Autodesk Fusion 360 part; units mm, degrees
(part 3 of 4)
sketch "Sketch2" plane through (0, 0, 0) normal (0, 1, 0) x (-1, 0, 0)
  line L0 (13, -8.25) -> (13, -4.1)
  line L1 (13, -4.1) -> (14, -4.1)
  line L2 (13, -4.1) -> (14, -4.1)
  line L3 (14, -4.1) -> (14, -5.1)
  line L4 (14, -5.1) -> (15, -5.1)
  line L5 (15, -5.1) -> (15, -13)
  line L6 (5.1, -15) -> (13, -15)
  line L7 (13, -15) -> (5.1, -15)
  line L8 (5.1, -14) -> (4.1, -14)
  line L9 (4.1, -14) -> (4.1, -13)
  line L10 (4.1, -13) -> (8.25, -13)
  arc A0 (13, -15) -> (15, -13) centre (13, -13) ccw
  line L11 (12.5, -13.5) -> (10.75, -13.5)
  line L12 (9.75, -12.5) -> (9.75, -10.75)
  line L13 (10.75, -9.75) -> (12.5, -9.75)
  line L14 (13.5, -10.75) -> (13.5, -12.5)
  arc A1 (12.5, -13.5) -> (13.5, -12.5) centre (12.5, -12.5) ccw
  line L15 (12.5, -12.5) -> (-13, 13)
  arc A2 (12.5, -13.5) -> (13.5, -12.5) centre (12.5, -12.5) ccw
  arc A3 (9.75, -12.5) -> (10.75, -13.5) centre (10.75, -12.5) ccw
  arc A4 (10.75, -9.75) -> (9.75, -10.75) centre (10.75, -10.75) ccw
  arc A5 (13.5, -10.75) -> (12.5, -9.75) centre (12.5, -10.75) ccw
  line L16 (15, -13) -> (15, -5.1)
  line L17 (12.5, -9.75) -> (10.75, -9.75)
  line L18 (10.75, -13.5) -> (12.5, -13.5)
  line L19 (9.5009, -9.5009) -> (1.6153, -1.6153) construction
  line L20 (8.25, -13) -> (8.25, -9.6642)
  line L21 (8.25, -10.6606) -> (8.25, -13)
  line L22 (13, -8.25) -> (9.6642, -8.25)
  line L23 (5.1, -14) -> (5.1, -15)
  line L24 (9.6642, -8.25) -> (5.5142, -4.1)
  line L25 (8.25, -9.6642) -> (4.1, -5.5142)
  line L26 (13.5, 10.75) -> (13.5, 12.5)
  arc A6 (13.5, 12.5) -> (12.5, 13.5) centre (12.5, 12.5) ccw
  arc A7 (10.75, 13.5) -> (9.75, 12.5) centre (10.75, 12.5) ccw
  line L27 (9.75, 12.5) -> (9.75, 10.75)
  line L28 (9.5009, 9.5009) -> (1.6153, 1.6153) construction
  line L29 (13, 8.25) -> (13, 4.1)
  arc A8 (9.75, 10.75) -> (10.75, 9.75) centre (10.75, 10.75) ccw
  line L30 (13, 4.1) -> (14, 4.1)
  arc A9 (13.5, 12.5) -> (12.5, 13.5) centre (12.5, 12.5) ccw
  line L31 (13, 4.1) -> (14, 4.1)
  line L32 (14, 4.1) -> (14, 5.1)
  line L33 (14, 5.1) -> (15, 5.1)
  line L34 (10.75, 9.75) -> (12.5, 9.75)
  line L35 (12.5, 9.75) -> (10.75, 9.75)
  line L36 (13, 8.25) -> (9.6642, 8.25)
  arc A10 (12.5, 9.75) -> (13.5, 10.75) centre (12.5, 10.75) ccw
  line L37 (4.1, 14) -> (4.1, 13)
  line L38 (5.1, 14) -> (4.1, 14)
  line L39 (15, 13) -> (15, 5.1)
  line L40 (15, 5.1) -> (15, 13)
  line L41 (5.1, 15) -> (13, 15)
  line L42 (13, 15) -> (5.1, 15)
  line L43 (4.1, 13) -> (8.25, 13)
  line L44 (12.5, 13.5) -> (10.75, 13.5)
  line L45 (10.75, 13.5) -> (12.5, 13.5)
  line L46 (8.25, 13) -> (8.25, 9.6642)
  line L47 (9.6642, 8.25) -> (5.5142, 4.1)
  line L48 (8.25, 10.6606) -> (8.25, 13)
  arc A11 (15, 13) -> (13, 15) centre (13, 13) ccw
  line L49 (8.25, 9.6642) -> (4.1, 5.5142)
  line L50 (5.1, 14) -> (5.1, 15)
  line L51 (-8.25, 9.6642) -> (-4.1, 5.5142)
  line L52 (-8.25, 10.6606) -> (-8.25, 13)
  line L53 (-12.5, -13.5) -> (-10.75, -13.5)
  arc A12 (-10.75, 9.75) -> (-9.75, 10.75) centre (-10.75, 10.75) ccw
  line L54 (-8.25, 13) -> (-8.25, 9.6642)
  line L55 (-4.1, -13) -> (-8.25, -13)
  line L56 (-15, -5.1) -> (-15, -13)
  line L57 (-9.75, 12.5) -> (-9.75, 10.75)
  line L58 (-13, -8.25) -> (-13, -4.1)
  line L59 (-8.25, -10.6606) -> (-8.25, -13)
  line L60 (-13, 8.25) -> (-13, 4.1)
  line L61 (-12.5, 13.5) -> (-10.75, 13.5)
  line L62 (-4.1, 13) -> (-8.25, 13)
  line L63 (-4.1, -14) -> (-4.1, -13)
  line L64 (-13, -15) -> (-5.1, -15)
  line L65 (-13.5, 10.75) -> (-13.5, 12.5)
  line L66 (-8.25, -13) -> (-8.25, -9.6642)
  line L67 (-9.6642, 8.25) -> (-5.5142, 4.1)
  arc A13 (-12.5, 13.5) -> (-13.5, 12.5) centre (-12.5, 12.5) ccw
  line L68 (-10.75, 13.5) -> (-12.5, 13.5)
  arc A14 (-13.5, -12.5) -> (-12.5, -13.5) centre (-12.5, -12.5) ccw
  line L69 (-13, -8.25) -> (-9.6642, -8.25)
  arc A15 (-12.5, -9.75) -> (-13.5, -10.75) centre (-12.5, -10.75) ccw
  arc A16 (-10.75, -13.5) -> (-9.75, -12.5) centre (-10.75, -12.5) ccw
  line L70 (-14, 5.1) -> (-15, 5.1)
  line L71 (-14, -5.1) -> (-15, -5.1)
  line L72 (-13, 15) -> (-5.1, 15)
  line L73 (-10.75, 9.75) -> (-12.5, 9.75)
  line L74 (-13, -4.1) -> (-14, -4.1)
  line L75 (-5.1, -14) -> (-5.1, -15)
  line L76 (-14, 4.1) -> (-14, 5.1)
  arc A17 (-9.75, -10.75) -> (-10.75, -9.75) centre (-10.75, -10.75) ccw
  line L77 (-14, -4.1) -> (-14, -5.1)
  line L78 (-15, 13) -> (-15, 5.1)
  line L79 (-10.75, -13.5) -> (-12.5, -13.5)
  line L80 (-13.5, -10.75) -> (-13.5, -12.5)
  line L81 (-5.1, -15) -> (-13, -15)
  arc A18 (-9.75, 12.5) -> (-10.75, 13.5) centre (-10.75, 12.5) ccw
  line L82 (-13, 4.1) -> (-14, 4.1)
  line L83 (-13, -4.1) -> (-14, -4.1)
  line L84 (-5.1, 14) -> (-5.1, 15)
  line L85 (-8.25, -9.6642) -> (-4.1, -5.5142)
  line L86 (-13, 4.1) -> (-14, 4.1)
  arc A19 (-13.5, 10.75) -> (-12.5, 9.75) centre (-12.5, 10.75) ccw
  line L87 (-15, -13) -> (-15, -5.1)
  line L88 (-9.5009, 9.5009) -> (-1.6152, 1.6153) construction
  line L89 (-10.75, -9.75) -> (-12.5, -9.75)
  line L90 (-5.1, 14) -> (-4.1, 14)
  line L91 (-15, 5.1) -> (-15, 13)
  line L92 (-9.75, -12.5) -> (-9.75, -10.75)
  arc A20 (-13, 15) -> (-15, 13) centre (-13, 13) ccw
  line L93 (-12.5, -9.75) -> (-10.75, -9.75)
  arc A21 (-15, -13) -> (-13, -15) centre (-13, -13) ccw
  arc A22 (-13.5, -12.5) -> (-12.5, -13.5) centre (-12.5, -12.5) ccw
  arc A23 (-12.5, 13.5) -> (-13.5, 12.5) centre (-12.5, 12.5) ccw
  line L94 (-5.1, -14) -> (-4.1, -14)
  line L95 (-12.5, 9.75) -> (-10.75, 9.75)
  line L96 (-9.5009, -9.5009) -> (-1.6152, -1.6153) construction
  line L97 (-5.1, 15) -> (-13, 15)
  line L98 (-13, 8.25) -> (-9.6642, 8.25)
  line L99 (-9.6642, -8.25) -> (-5.5142, -4.1)
  line L100 (-4.1, 14) -> (-4.1, 13)
  line L101 (4.1, -5.5142) -> (-4.1, -5.5142)
  line L102 (5.5142, 4.1) -> (5.5142, -4.1)
  line L103 (-5.5142, 4.1) -> (-5.5142, -4.1)
  line L104 (4.1, 5.5142) -> (-4.1, 5.5142)
  circle A24 centre (0, 0) radius 3.4
  point P0 (13, -8.25)
  point P1 (14, -4.1)
  point P2 (14, -5.1)
  point P3 (15, -5.1)
  point P4 (15, -15)
  point P5 (5.1, -15)
  point P6 (5.1, -14)
  point P7 (4.1, -14)
  point P8 (4.1, -13)
  point P9 (8.25, -13)
  point P10 (0, 0)
  point P11 (15, 0)
  point P12 (0, 15)
  point P13 (0, 0)
  point P14 (15, 15)
  point P15 (12.5, 12.5)
  point P16 (5.1, 14)
  point P17 (5.1, 15)
  point P18 (8.25, 13)
  point P19 (4.1, 13)
  point P20 (14, 5.1)
  point P21 (4.1, 14)
  point P22 (14, 4.1)
  point P23 (13, 8.25)
  point P24 (15, 5.1)
  point P25 (-12.5, 12.5)
  point P26 (-15, 0)
  point P27 (-5.1, 15)
  point P28 (-8.25, 13)
  point P29 (-4.1, 13)
  point P30 (-5.1, -15)
  point P31 (-15, 15)
  point P32 (-14, 5.1)
  point P33 (-4.1, 14)
  point P34 (-14, 4.1)
  point P35 (-13, 8.25)
  point P36 (-15, 5.1)
  point P37 (-4.1, -13)
  point P38 (0, 0)
  point P39 (0, 0)
  point P40 (0, 15)
  point P41 (0, 15)
  point P42 (0, -15)
  point P43 (0, 0)
  point P44 (-8.25, -13)
  point P45 (-4.1, -14)
  point P46 (-15, -15)
  point P47 (-5.1, -14)
  point P48 (-12.5, -12.5)
  point P49 (0, 0)
  point P50 (-5.1, 14)
  point P51 (-15, -5.1)
  point P52 (-14, -5.1)
  point P53 (-13, -8.25)
  point P54 (-14, -4.1)
  point P55 (-15, 0)
  dimension "d78" = 2
  dimension "d79" = 1
  dimension "d80" = 1.5
  dimension "d91" = 1
  dimension "d92" = 1
  dimension "d93" = 1.5
  dimension "d94" = 1.5
  dimension "d102" = 3.75
  dimension "d103" = 1.5
  dimension "d104" = 3.75
  dimension "d105" = 2
  dimension "d106" = 2
  dimension "d109" = 5.869
  dimension "d110" = 5.869
  dimension "d111" = 3.3358
  dimension "d112" = 3.3358
  dimension "d113" = 4.15
  dimension "d114" = 4.15
  dimension "d115" = 8.2
  dimension "d116" = 8.2
  dimension "d117" = 8.2
  dimension "d118" = 8.2
  dimension "d119" = 6.8
  constraint coincident L0.end L1.start
  constraint coincident P1 L1.end
  constraint coincident P2 L3.end
  constraint coincident P3 L4.end
  constraint coincident P5 L6.start
  constraint coincident P6 L8.start
  constraint coincident P7 L8.end
  constraint coincident P8 L9.end
  constraint coincident P9 L10.end
  constraint tangent L5 A0
  constraint tangent L7 A0
  constraint horizontal L11
  constraint vertical L12
  constraint horizontal L13
  constraint vertical L14
  constraint tangent L14 A2
  constraint tangent L11 A2
  constraint tangent L11 A3
  constraint tangent L12 A3
  constraint equal A2 A3
  constraint tangent L12 A4
  constraint tangent L13 A4
  constraint equal A2 A4
  constraint tangent L13 A5
  constraint tangent L14 A5
  constraint equal A2 A5
  constraint coincident L15 L19.start
  constraint coincident L15 L19.end
  constraint parallel L15 L19
  constraint perpendicular L10 L20
  constraint coincident P0 L0.start
  constraint perpendicular L0 L22
  constraint parallel L19 L24
  constraint parallel L19 L25
  constraint perpendicular L7 L23
  constraint coincident P49 P43
  measures "d78" radius of A0
  measures "d79" radius of A2
  measures "d80" distance of L14 L16
  measures "d91" distance of L19 L24
  measures "d92" distance of L15 L25
  measures "d93" distance of L12 L20
  measures "d94" distance of L13 L22
  measures "d102" distance of L12 L14
  measures "d103" distance of L7 L11
  measures "d104" distance of L11 L13
  measures "d105" distance of L7 L10
  measures "d106" distance of L0 L5
  measures "d109" distance of L22.end L24.end
  measures "d110" distance of L20.end L25.end
  measures "d111" distance of P9 L20.end
  measures "d112" distance of P0 L22.end
  measures "d113" distance of P8 P9
  measures "d114" distance of P0 L0.end
  measures "d115" distance of L25.end L85.end
  measures "d116" distance of L24.end L47.end
  measures "d117" distance of L67.end L99.end
  measures "d118" distance of L49.end L51.end
  measures "d119" diameter of A24
extrude "Extrude1" add sketch "Sketch2" along normal blind 100
move_body "Move1" bodies 1 to x (0, -1, 0) y (1, 0, 0) z (0, 0, 1) at (-3.4, 15.1, 15)
move_body "Move2" bodies 1 to x (1, 0, 0) y (0, 1, 0) z (0, 0, 1) at (3.4, 0, 0)
sketch "Sketch3" plane through (0, 0, 30) normal (0, 0, 1) x (1, 0, 0)
  line L0 (0, 10) -> (0, 2.1)
  line L1 (0, 2.1) -> (100, 2.1)
  line L2 (100, 2.1) -> (100, 10)
  line L3 (100, 10) -> (0, 10)
  line L4 (0, 0) -> (64.1772, 37.0527)
  line L5 (0, 0) -> (74.1054, 0) construction
  line L6 (64.1772, 37.0527) -> (-5, 37.0527)
  line L7 (-5, 37.0527) -> (-5, 0)
  line L8 (-5, 0) -> (0, 0)
  line L9 (100, 30) -> (54.3421, 30) construction
  line L10 (100, 0) -> (78.7466, 36.812)
  line L11 (100, 0) -> (57.4932, 0) construction
  line L12 (78.7466, 36.812) -> (120, 36.812)
  line L13 (120, 36.812) -> (120, -10)
  line L14 (120, -10) -> (99.3733, -10)
  line L15 (99.3733, -10) -> (100, 0)
  dimension "d122" = 30
  dimension "d126" = 60
  constraint horizontal L5
  constraint coincident L4.start L5.start
  constraint horizontal L6
  constraint perpendicular L6 L7
  constraint perpendicular L7 L8
  constraint horizontal L9
  constraint horizontal L11
  constraint parallel L3 L12
  constraint perpendicular L3 L13
  constraint perpendicular L13 L14
  measures "d122" angle of L4 L5
  measures "d126" angle of L10 L11
extrude "Extrude2" cut sketch "Sketch3" against normal blind 60 contours L0 L1 L3 L4 | L0 L1 L3 L4 L6 L7 L8 | L1 L2 L3 L10 L12 L13 L14 L15 | L1 L2 L3 L10
equation "d33 = ( 8.2 / 2 ) * 1 mm"
equation "d59 = ( 8.5 / 2 ) * 1 mm"
equation "d60 = ( 8.5 / 2 ) * 1 mm"
equation "d72 = ( 8.2 / 2 ) * 1 mm"
equation "Length = 100 mm"

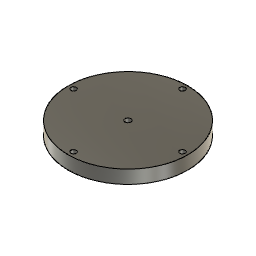
design "lidar_holder"
Autodesk Fusion 360 part; units mm, degrees
sketch "Sketch1" plane through (0, 0, 0) normal (0, 0, 1) x (1, 0, 0)
  circle A0 centre (0, 0) radius 45
  circle A1 centre (-41, 0) radius 2
  circle A2 centre (0, -41) radius 2
  circle A3 centre (41, 0) radius 2
  circle A4 centre (0, 41) radius 2
  circle A5 centre (0, 0) radius 2.25
  dimension "d1" = 90
  dimension "d2" = 4
  dimension "d4" = 4
  dimension "d5" = 4
  dimension "d6" = 4
  dimension "d7" = 4.5
  constraint coincident A0.centre A5.centre
  measures "d1" diameter of A0
  measures "d2" diameter of A1
  measures "d4" diameter of A2
  measures "d5" diameter of A3
  measures "d6" diameter of A4
  measures "d7" diameter of A5
extrude "Extrude1" add sketch "Sketch1" along normal blind 10

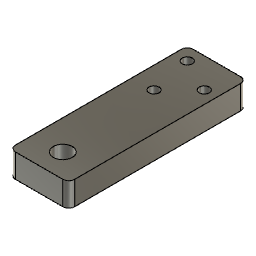
design "wheel_holder"
Autodesk Fusion 360 part; units mm, degrees
sketch "Sketch1" plane through (0, 0, 0) normal (0, 0, 1) x (1, 0, 0)
  line L0 (0, 0) -> (50, 0)
  line L1 (50, 0) -> (50, 150)
  line L2 (50, 150) -> (0, 150)
  line L3 (0, 150) -> (0, 0)
  dimension "d1" = 150
  dimension "d2" = 50
  constraint horizontal L0
  constraint vertical L1
  constraint horizontal L2
  constraint vertical L3
  constraint coincident L0.start L3.end
  measures "d1" distance of L0.start L2.end
  measures "d2" distance of L0.start L0.end
extrude "Extrude1" add sketch "Sketch1" along normal blind 20
fillet "Fillet1" radius 5 4 edges at (0, 0, 10) (50, 0, 10) (50, 150, 10) (0, 150, 10)
sketch "Sketch2" plane through (0, 0, 20) normal (0, 0, 1) x (-1, 0, 0)
  arc A0 (-5, -150) -> (0, -145) centre (-5, -145) ccw
  line L0 (0, -145) -> (0, -5)
  arc A1 (0, -5) -> (-5, 0) centre (-5, -5) ccw
  line L1 (-5, 0) -> (-45, 0)
  arc A2 (-45, 0) -> (-50, -5) centre (-45, -5) ccw
  line L2 (-50, -5) -> (-50, -145)
  arc A3 (-50, -145) -> (-45, -150) centre (-45, -145) ccw
  line L3 (-45, -150) -> (-5, -150)
  circle A4 centre (-25, -20) radius 8
  circle A5 centre (-39.3934, -125) radius 4.25
  circle A6 centre (-18.1802, -103.8009) radius 4.25
  circle A7 centre (-11.0104, -138.9896) radius 4.25
  dimension "d6" = 16
  dimension "d7" = 20
  dimension "d10" = 8.5
  dimension "d13" = 8.5
  dimension "d19" = 8.5
  dimension "d26" = 8.5
  measures "d6" diameter of A4
  measures "d7" distance of L1 A4.centre
  measures "d10" diameter of A5
  measures "d13" diameter of A6
  measures "d19" diameter of A7
  measures "d26" distance of A0.centre A7.centre
extrude "Extrude2" cut sketch "Sketch2" against normal blind 60 contours A4 | A5 | A6 | A7

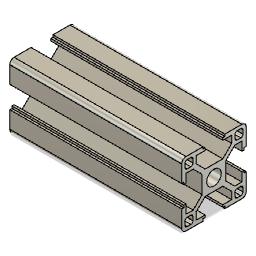
design "tslot_80mm"
Autodesk Fusion 360 part; units mm, degrees
sketch "Sketch1" plane through (0, 0, 0) normal (0, 1, 0) x (1, 0, 0)
  circle A0 centre (0, 0) radius 3.4
  line L0 (5.8, -4.25) -> (5.8, 4.25)
  line L1 (4.4302, 5.8) -> (-4.0698, 5.8)
  line L2 (-5.8, 4.25) -> (-5.8, -4.25)
  arc A1 (-13, 15) -> (-15, 13) centre (-13, 13) ccw
  arc A2 (15, 13) -> (13, 15) centre (13, 13) ccw
  arc A3 (12.9984, -15) -> (15, -13) centre (13, -13) ccw
  arc A4 (-15, -13.001) -> (-13, -15) centre (-13, -13) ccw
  line L3 (-9.0785, 8.25) -> (-13, 8.25)
  line L4 (-10.4448, -8.25) -> (-13, -8.25)
  line L5 (-8.25, 10.6606) -> (-8.25, 13)
  line L6 (8.25, 9.241) -> (8.25, 13)
  line L7 (-12.5, 9.75) -> (-10.75, 9.75)
  line L8 (-9.75, 10.75) -> (-9.75, 12.5)
  line L9 (-10.75, 13.5) -> (-12.5, 13.5)
  line L10 (-13.5, 12.5) -> (-13.5, 10.75)
  arc A5 (-12.5, 13.5) -> (-13.5, 12.5) centre (-12.5, 12.5) ccw
  arc A6 (-9.75, 12.5) -> (-10.75, 13.5) centre (-10.75, 12.5) ccw
  arc A7 (-10.75, 9.75) -> (-9.75, 10.75) centre (-10.75, 10.75) ccw
  arc A8 (-13.5, 10.75) -> (-12.5, 9.75) centre (-12.5, 10.75) ccw
  line L11 (-4.1, 14) -> (-5.1, 14)
  line L12 (-5.1, 14) -> (-5.1, 15)
  line L13 (4.1, 13) -> (4.1, 14)
  line L14 (4.1, 14) -> (5.1, 14)
  line L15 (5.1, 14) -> (5.1, 15)
  line L16 (-4.1, 14) -> (-4.1, 13)
  line L17 (0, 15) -> (0, -15) construction
  line L18 (-15, 0) -> (15, 0) construction
  line L19 (13.5, 12.5) -> (13.5, 10.75)
  line L20 (12.5, 9.75) -> (10.75, 9.75)
  arc A9 (10.75, 13.5) -> (9.75, 12.5) centre (10.75, 12.5) ccw
  arc A10 (9.75, 10.75) -> (10.75, 9.75) centre (10.75, 10.75) ccw
  line L21 (9.75, 10.75) -> (9.75, 12.5)
  arc A11 (12.5, 9.75) -> (13.5, 10.75) centre (12.5, 10.75) ccw
  line L22 (10.75, 13.5) -> (12.5, 13.5)
  arc A12 (13.5, 12.5) -> (12.5, 13.5) centre (12.5, 12.5) ccw
  arc A13 (-9.75, -10.75) -> (-10.75, -9.75) centre (-10.75, -10.75) ccw
  line L23 (-9.75, -10.75) -> (-9.75, -12.5)
  line L24 (-13.5, -12.5) -> (-13.5, -10.75)
  line L25 (-10.75, -13.5) -> (-12.5, -13.5)
  arc A14 (-13.5, -12.5) -> (-12.5, -13.5) centre (-12.5, -12.5) ccw
  line L26 (-12.5, -9.75) -> (-10.75, -9.75)
  arc A15 (-12.5, -9.75) -> (-13.5, -10.75) centre (-12.5, -10.75) ccw
  arc A16 (-10.75, -13.5) -> (-9.75, -12.5) centre (-10.75, -12.5) ccw
  arc A17 (12.5, -13.5) -> (13.5, -12.5) centre (12.5, -12.5) ccw
  arc A18 (10.75, -9.75) -> (9.75, -10.75) centre (10.75, -10.75) ccw
  arc A19 (9.75, -12.5) -> (10.75, -13.5) centre (10.75, -12.5) ccw
  line L27 (9.75, -10.75) -> (9.75, -12.5)
  line L28 (12.5, -9.75) -> (10.75, -9.75)
  arc A20 (13.5, -10.75) -> (12.5, -9.75) centre (12.5, -10.75) ccw
  line L29 (13.5, -12.5) -> (13.5, -10.75)
  line L30 (10.75, -13.5) -> (12.5, -13.5)
  line L31 (-4.1, -14) -> (-5.1, -14)
  line L32 (-4.1, -14) -> (-4.1, -13)
  line L33 (-5.1, -14) -> (-5.1, -15)
  line L34 (4.1, -13) -> (4.1, -14)
  line L35 (4.1, -14) -> (5.1, -14)
  line L36 (5.1, -14) -> (5.1, -15)
  line L37 (-8.25, -10.6606) -> (-8.25, -13)
  line L38 (-13, -15) -> (-5.1, -15)
  line L39 (5.1, -15) -> (12.9984, -15)
  line L40 (-8.25, -13) -> (-4.1, -13)
  line L41 (13, 15) -> (5.1, 15)
  line L42 (-5.1, 15) -> (-13, 15)
  line L43 (8.25, 13) -> (4.1, 13)
  line L44 (-4.1, 13) -> (-8.25, 13)
  line L45 (8.25, -9.768) -> (8.25, -13)
  line L46 (-13, -13) -> (12.5, 12.5) construction
  line L47 (-12.5, 12.5) -> (13, -13) construction
  line L48 (13, -8.25) -> (9.8438, -8.25)
  line L49 (5.8, -4.25) -> (9.8438, -8.25)
  line L50 (4.1, -13) -> (8.25, -13)
  line L51 (13, 8.25) -> (9.3051, 8.25)
  line L52 (-4.2601, -5.7908) -> (4.2399, -5.7908)
  line L53 (-13, 4.1) -> (-14, 4.1)
  line L54 (-14, 4.1) -> (-14, 5.1)
  line L55 (-14, 5.1) -> (-15, 5.1)
  line L56 (-13, -4.1) -> (-14, -4.1)
  line L57 (-14, -4.1) -> (-14, -5.1)
  line L58 (-14, -5.1) -> (-15, -5.1)
  line L59 (-13, 8.25) -> (-13, 4.1)
  line L60 (-13, -4.1) -> (-13, -8.25)
  line L61 (-15, 13) -> (-15, 5.1)
  line L62 (-15, -5.1) -> (-15, -13.001)
  line L63 (13, -8.25) -> (13, -3.9838)
  line L64 (13, 4.0895) -> (13, 10.5589)
  line L65 (15, -13) -> (15, -4.9838)
  line L66 (15, 5.0895) -> (15, 13)
  point P0 (15, -15)
  point P1 (15, 15)
  point P2 (-15, 15)
  point P3 (13, 13)
  point P4 (-13, -13)
  point P5 (13, -13)
  point P6 (13, -13)
  point P7 (13, -10.5589)
  dimension "d1" = 6.8
  dimension "d2" = 30
  dimension "d3" = 30
  dimension "d5" = 9.2
  dimension "d6" = 9.2
  dimension "d7" = 9.2
  dimension "d13" = 2
  dimension "d14" = 2
  dimension "d15" = 2
  dimension "d16" = 2
  dimension "d17" = 16.5
  dimension "d19" = 16.5
  dimension "d22" = 1.5
  dimension "d23" = 1.5
  dimension "d24" = 1.5
  dimension "d25" = 1.5
  dimension "d26" = 1
  dimension "d33" = 4.1
  dimension "d34" = 1
  dimension "d35" = 2
  dimension "d36" = 2
  dimension "d37" = 2
  dimension "d39" = 3.75
  dimension "d40" = 3.75
  dimension "d41" = 5.8
  dimension "d42" = 5.8
  dimension "d43" = 5.8
  dimension "d45" = 8.5
  dimension "d46" = 8.5
  dimension "d48" = 8.5
  dimension "d49" = 1
  dimension "d51" = 8.2
  dimension "d52" = 1.5
  dimension "d53" = 1.5
  dimension "d54" = 1.5
  dimension "d55" = 1.5
  dimension "d57" = 1.5
  dimension "d58" = 1.5
  dimension "d59" = 4.25
  dimension "d60" = 4.25
  dimension "d64" = 8.5
  dimension "d65" = 1
  dimension "d66" = 1
  dimension "d67" = 1
  dimension "d68" = 1
  dimension "d71" = 8.2
  dimension "d72" = 4.1
  constraint horizontal L38
  constraint vertical L65
  constraint horizontal L41
  constraint vertical L61
  constraint vertical L0
  constraint horizontal L1
  constraint vertical L2
  constraint coincident P2 L61
  constraint coincident P2 L41
  constraint tangent A1 L61
  constraint coincident P1 L41
  constraint coincident P1 L65
  constraint tangent A2 L41
  constraint coincident P0 L38
  constraint coincident P0 L65
  constraint tangent A3 L65
  constraint tangent A4 L38
  constraint parallel L63 L65
  constraint horizontal L7
  constraint vertical L8
  constraint horizontal L9
  constraint vertical L10
  constraint tangent L10 A5
  constraint tangent L9 A5
  constraint tangent L9 A6
  constraint tangent L8 A6
  constraint equal A5 A6
  constraint tangent L8 A7
  constraint tangent L7 A7
  constraint equal A5 A7
  constraint tangent L7 A8
  constraint tangent L10 A8
  constraint equal A5 A8
  constraint perpendicular L12 L41
  constraint perpendicular L13 L43
  constraint perpendicular L13 L14
  constraint perpendicular L15 L41
  constraint coincident L16.end L43
  constraint perpendicular L16 L43
  constraint symmetric A1.centre L17 P3
  constraint symmetric L10.start L17 L19.start
  constraint symmetric L9.end L17 L22.end
  constraint symmetric A5 L17 A12
  constraint symmetric L9.start L17 A9.start
  constraint symmetric L8.end L17 A9.end
  constraint symmetric A6 L17 A9
  constraint symmetric L8.start L17 A10.start
  constraint symmetric L7.end L17 L20.end
  constraint symmetric A7 L17 A10
  constraint symmetric L7.start L17 L20.start
  constraint symmetric L10.end L17 L19.end
  constraint symmetric A8 L17 A11
  constraint symmetric P3 L18 P6
  constraint symmetric L64.end L18 P7
  constraint symmetric L18 L19.end A20.start
  constraint symmetric L18 L20.end A18.start
  constraint symmetric L18 P3 P6
  constraint symmetric L18 L19.start A17.end
  constraint symmetric L18 L22.end A17.start
  constraint symmetric L18 A9.end A19.start
  constraint symmetric L18 L20.start L28.start
  constraint symmetric L18 A10.start A18.end
  constraint symmetric L18 A9.start A19.end
  constraint symmetric L18 A9 A19
  constraint symmetric L18 A10 A18
  constraint symmetric L18 A11 A20
  constraint symmetric L18 A12 A17
  constraint symmetric L5.end L18 L37.end
  constraint symmetric L11.start L18 L31.start
  constraint symmetric L11.end L18 L31.end
  constraint symmetric L12.end L18 L33.end
  constraint symmetric L13.start L18 L34.start
  constraint symmetric L13.end L18 L34.end
  constraint symmetric L14.end L18 L35.end
  constraint symmetric L15.end L18 L36.end
  constraint symmetric L16.end L18 L32.end
  constraint collinear L38 L39
  constraint collinear L41 L42
  constraint collinear L43 L44
  constraint symmetric L17 L37.end L45.end
  constraint coincident P4 A4.centre
  constraint coincident A12.centre L46.end
  constraint coincident A5.centre L47.start
  constraint coincident P6 P5
  constraint perpendicular L48 L63
  constraint vertical L45
  constraint coincident L51.start L63
  constraint horizontal L52
  constraint coincident L56.start L59
  constraint coincident L58.end L61
  constraint collinear L59 L60
  constraint collinear L61 L62
  constraint perpendicular L53 L54
  constraint perpendicular L54 L55
  constraint perpendicular L57 L58
  constraint perpendicular L56 L57
  constraint perpendicular L58 L62
  constraint collinear L65 L66
  measures "d1" diameter of A0
  measures "d2" distance of P0 P1
  measures "d3" distance of P1 P2
  measures "d5" distance of L0 L65
  measures "d6" distance of L2 L61
  measures "d7" distance of L1 L41
  measures "d13" radius of A1
  measures "d14" radius of A2
  measures "d15" radius of A3
  measures "d16" radius of A4
  measures "d17" distance of L3 L4
  measures "d19" distance of L5 L6
  measures "d22" distance of L5 L8
  measures "d23" distance of L10 L61
  measures "d24" distance of L3 L7
  measures "d25" distance of L9 L41
  measures "d26" radius of A5
  measures "d33" distance of A0.centre L13
  measures "d34" distance of L11.start L11.end
  measures "d35" distance of L41 L43
  measures "d36" distance of L59 L61
  measures "d37" distance of L63 L65
  measures "d39" distance of L8 L10
  measures "d40" distance of L7 L9
  measures "d41" distance of A0.centre L1
  measures "d42" distance of A0.centre L2
  measures "d43" distance of A0.centre L0
  measures "d45" distance of L1.end L1.start
  measures "d46" distance of L2.start L2.end
  measures "d48" distance of L0.start L0.end
  measures "d49" distance of L13.end L14.end
  measures "d51" distance of L13 L16
  measures "d52" distance of L23 L37
  measures "d53" distance of L4 L26
  measures "d54" distance of L27 L45
  measures "d55" distance of L28 L48
  measures "d57" distance of L20 L51
  measures "d58" distance of L6 L21
  measures "d59" distance of L2.end L18
  measures "d60" distance of L0.start L18
  measures "d64" distance of L52.start L52.end
  measures "d65" distance of L53.end L54.end
  measures "d66" distance of L53.start L53.end
  measures "d67" distance of L56.start L56.end
  measures "d68" distance of L56.end L57.end
  measures "d71" distance of L53 L56
  measures "d72" distance of L18 L53
sketch "Sketch2" plane through (0, 0, 0) normal (0, 1, 0) x (-1, 0, 0)
  line L0 (13, -8.25) -> (13, -4.1)
  line L1 (13, -4.1) -> (14, -4.1)
  line L2 (13, -4.1) -> (14, -4.1)
  line L3 (14, -4.1) -> (14, -5.1)
  line L4 (14, -5.1) -> (15, -5.1)
  line L5 (15, -5.1) -> (15, -13)
  line L6 (5.1, -15) -> (13, -15)
  line L7 (13, -15) -> (5.1, -15)
  line L8 (5.1, -14) -> (4.1, -14)
  line L9 (4.1, -14) -> (4.1, -13)
  line L10 (4.1, -13) -> (8.25, -13)
  arc A0 (13, -15) -> (15, -13) centre (13, -13) ccw
  line L11 (12.5, -13.5) -> (10.75, -13.5)
  line L12 (9.75, -12.5) -> (9.75, -10.75)
  line L13 (10.75, -9.75) -> (12.5, -9.75)
  line L14 (13.5, -10.75) -> (13.5, -12.5)
  arc A1 (12.5, -13.5) -> (13.5, -12.5) centre (12.5, -12.5) ccw
  line L15 (12.5, -12.5) -> (-13, 13)
  arc A2 (12.5, -13.5) -> (13.5, -12.5) centre (12.5, -12.5) ccw
  arc A3 (9.75, -12.5) -> (10.75, -13.5) centre (10.75, -12.5) ccw
  arc A4 (10.75, -9.75) -> (9.75, -10.75) centre (10.75, -10.75) ccw
  arc A5 (13.5, -10.75) -> (12.5, -9.75) centre (12.5, -10.75) ccw
  line L16 (15, -13) -> (15, -5.1)
  line L17 (12.5, -9.75) -> (10.75, -9.75)
  line L18 (10.75, -13.5) -> (12.5, -13.5)
  line L19 (9.5009, -9.5009) -> (1.6153, -1.6153) construction
  line L20 (8.25, -13) -> (8.25, -9.6642)
  line L21 (8.25, -10.6606) -> (8.25, -13)
  line L22 (13, -8.25) -> (9.6642, -8.25)
  line L23 (5.1, -14) -> (5.1, -15)
  line L24 (9.6642, -8.25) -> (5.5142, -4.1)
  line L25 (8.25, -9.6642) -> (4.1, -5.5142)
  line L26 (13.5, 10.75) -> (13.5, 12.5)
  arc A6 (13.5, 12.5) -> (12.5, 13.5) centre (12.5, 12.5) ccw
  arc A7 (10.75, 13.5) -> (9.75, 12.5) centre (10.75, 12.5) ccw
  line L27 (9.75, 12.5) -> (9.75, 10.75)
  line L28 (9.5009, 9.5009) -> (1.6153, 1.6153) construction
  line L29 (13, 8.25) -> (13, 4.1)
  arc A8 (9.75, 10.75) -> (10.75, 9.75) centre (10.75, 10.75) ccw
  line L30 (13, 4.1) -> (14, 4.1)
  arc A9 (13.5, 12.5) -> (12.5, 13.5) centre (12.5, 12.5) ccw
  line L31 (13, 4.1) -> (14, 4.1)
  line L32 (14, 4.1) -> (14, 5.1)
  line L33 (14, 5.1) -> (15, 5.1)
  line L34 (10.75, 9.75) -> (12.5, 9.75)
  line L35 (12.5, 9.75) -> (10.75, 9.75)
  line L36 (13, 8.25) -> (9.6642, 8.25)
  arc A10 (12.5, 9.75) -> (13.5, 10.75) centre (12.5, 10.75) ccw
  line L37 (4.1, 14) -> (4.1, 13)
  line L38 (5.1, 14) -> (4.1, 14)
  line L39 (15, 13) -> (15, 5.1)
  line L40 (15, 5.1) -> (15, 13)
  line L41 (5.1, 15) -> (13, 15)
  line L42 (13, 15) -> (5.1, 15)
  line L43 (4.1, 13) -> (8.25, 13)
  line L44 (12.5, 13.5) -> (10.75, 13.5)
  line L45 (10.75, 13.5) -> (12.5, 13.5)
  line L46 (8.25, 13) -> (8.25, 9.6642)
  line L47 (9.6642, 8.25) -> (5.5142, 4.1)
  line L48 (8.25, 10.6606) -> (8.25, 13)
  arc A11 (15, 13) -> (13, 15) centre (13, 13) ccw
  line L49 (8.25, 9.6642) -> (4.1, 5.5142)
  line L50 (5.1, 14) -> (5.1, 15)
  line L51 (-8.25, 9.6642) -> (-4.1, 5.5142)
  line L52 (-8.25, 10.6606) -> (-8.25, 13)
  line L53 (-12.5, -13.5) -> (-10.75, -13.5)
  arc A12 (-10.75, 9.75) -> (-9.75, 10.75) centre (-10.75, 10.75) ccw
  line L54 (-8.25, 13) -> (-8.25, 9.6642)
  line L55 (-4.1, -13) -> (-8.25, -13)
  line L56 (-15, -5.1) -> (-15, -13)
  line L57 (-9.75, 12.5) -> (-9.75, 10.75)
  line L58 (-13, -8.25) -> (-13, -4.1)
  line L59 (-8.25, -10.6606) -> (-8.25, -13)
  line L60 (-13, 8.25) -> (-13, 4.1)
  line L61 (-12.5, 13.5) -> (-10.75, 13.5)
  line L62 (-4.1, 13) -> (-8.25, 13)
  line L63 (-4.1, -14) -> (-4.1, -13)
  line L64 (-13, -15) -> (-5.1, -15)
  line L65 (-13.5, 10.75) -> (-13.5, 12.5)
  line L66 (-8.25, -13) -> (-8.25, -9.6642)
  line L67 (-9.6642, 8.25) -> (-5.5142, 4.1)
  arc A13 (-12.5, 13.5) -> (-13.5, 12.5) centre (-12.5, 12.5) ccw
  line L68 (-10.75, 13.5) -> (-12.5, 13.5)
  arc A14 (-13.5, -12.5) -> (-12.5, -13.5) centre (-12.5, -12.5) ccw
  line L69 (-13, -8.25) -> (-9.6642, -8.25)
  arc A15 (-12.5, -9.75) -> (-13.5, -10.75) centre (-12.5, -10.75) ccw
  arc A16 (-10.75, -13.5) -> (-9.75, -12.5) centre (-10.75, -12.5) ccw
  line L70 (-14, 5.1) -> (-15, 5.1)
  line L71 (-14, -5.1) -> (-15, -5.1)
  line L72 (-13, 15) -> (-5.1, 15)
  line L73 (-10.75, 9.75) -> (-12.5, 9.75)
  line L74 (-13, -4.1) -> (-14, -4.1)
  line L75 (-5.1, -14) -> (-5.1, -15)
  line L76 (-14, 4.1) -> (-14, 5.1)
  arc A17 (-9.75, -10.75) -> (-10.75, -9.75) centre (-10.75, -10.75) ccw
  line L77 (-14, -4.1) -> (-14, -5.1)
  line L78 (-15, 13) -> (-15, 5.1)
  line L79 (-10.75, -13.5) -> (-12.5, -13.5)
  line L80 (-13.5, -10.75) -> (-13.5, -12.5)
  line L81 (-5.1, -15) -> (-13, -15)
  arc A18 (-9.75, 12.5) -> (-10.75, 13.5) centre (-10.75, 12.5) ccw
  line L82 (-13, 4.1) -> (-14, 4.1)
  line L83 (-13, -4.1) -> (-14, -4.1)
  line L84 (-5.1, 14) -> (-5.1, 15)
  line L85 (-8.25, -9.6642) -> (-4.1, -5.5142)
  line L86 (-13, 4.1) -> (-14, 4.1)
  arc A19 (-13.5, 10.75) -> (-12.5, 9.75) centre (-12.5, 10.75) ccw
  line L87 (-15, -13) -> (-15, -5.1)
  line L88 (-9.5009, 9.5009) -> (-1.6152, 1.6153) construction
  line L89 (-10.75, -9.75) -> (-12.5, -9.75)
  line L90 (-5.1, 14) -> (-4.1, 14)
  line L91 (-15, 5.1) -> (-15, 13)
  line L92 (-9.75, -12.5) -> (-9.75, -10.75)
  arc A20 (-13, 15) -> (-15, 13) centre (-13, 13) ccw
  line L93 (-12.5, -9.75) -> (-10.75, -9.75)
  arc A21 (-15, -13) -> (-13, -15) centre (-13, -13) ccw
  arc A22 (-13.5, -12.5) -> (-12.5, -13.5) centre (-12.5, -12.5) ccw
  arc A23 (-12.5, 13.5) -> (-13.5, 12.5) centre (-12.5, 12.5) ccw
  line L94 (-5.1, -14) -> (-4.1, -14)
  line L95 (-12.5, 9.75) -> (-10.75, 9.75)
  line L96 (-9.5009, -9.5009) -> (-1.6152, -1.6153) construction
  line L97 (-5.1, 15) -> (-13, 15)
  line L98 (-13, 8.25) -> (-9.6642, 8.25)
  line L99 (-9.6642, -8.25) -> (-5.5142, -4.1)
  line L100 (-4.1, 14) -> (-4.1, 13)
  line L101 (4.1, -5.5142) -> (-4.1, -5.5142)
  line L102 (5.5142, 4.1) -> (5.5142, -4.1)
  line L103 (-5.5142, 4.1) -> (-5.5142, -4.1)
  line L104 (4.1, 5.5142) -> (-4.1, 5.5142)
  circle A24 centre (0, 0) radius 3.4
  point P0 (13, -8.25)
  point P1 (14, -4.1)
  point P2 (14, -5.1)
  point P3 (15, -5.1)
  point P4 (15, -15)
  point P5 (5.1, -15)
  point P6 (5.1, -14)
  point P7 (4.1, -14)
  point P8 (4.1, -13)
  point P9 (8.25, -13)
  point P10 (0, 0)
  point P11 (15, 0)
  point P12 (0, 15)
  point P13 (0, 0)
  point P14 (15, 15)
  point P15 (12.5, 12.5)
  point P16 (5.1, 14)
  point P17 (5.1, 15)
  point P18 (8.25, 13)
  point P19 (4.1, 13)
  point P20 (14, 5.1)
  point P21 (4.1, 14)
  point P22 (14, 4.1)
  point P23 (13, 8.25)
  point P24 (15, 5.1)
  point P25 (-12.5, 12.5)
  point P26 (-15, 0)
  point P27 (-5.1, 15)
  point P28 (-8.25, 13)
  point P29 (-4.1, 13)
  point P30 (-5.1, -15)
  point P31 (-15, 15)
  point P32 (-14, 5.1)
  point P33 (-4.1, 14)
  point P34 (-14, 4.1)
  point P35 (-13, 8.25)
  point P36 (-15, 5.1)
  point P37 (-4.1, -13)
  point P38 (0, 0)
  point P39 (0, 0)
  point P40 (0, 15)
  point P41 (0, 15)
  point P42 (0, -15)
  point P43 (0, 0)
  point P44 (-8.25, -13)
  point P45 (-4.1, -14)
  point P46 (-15, -15)
  point P47 (-5.1, -14)
  point P48 (-12.5, -12.5)
  point P49 (0, 0)
  point P50 (-5.1, 14)
  point P51 (-15, -5.1)
  point P52 (-14, -5.1)
  point P53 (-13, -8.25)
  point P54 (-14, -4.1)
  point P55 (-15, 0)
  dimension "d78" = 2
  dimension "d79" = 1
  dimension "d80" = 1.5
  dimension "d91" = 1
  dimension "d92" = 1
  dimension "d93" = 1.5
  dimension "d94" = 1.5
  dimension "d102" = 3.75
  dimension "d103" = 1.5
  dimension "d104" = 3.75
  dimension "d105" = 2
  dimension "d106" = 2
  dimension "d109" = 5.869
  dimension "d110" = 5.869
  dimension "d111" = 3.3358
  dimension "d112" = 3.3358
  dimension "d113" = 4.15
  dimension "d114" = 4.15
  dimension "d115" = 8.2
  dimension "d116" = 8.2
  dimension "d117" = 8.2
  dimension "d118" = 8.2
  dimension "d119" = 6.8
  constraint coincident L0.end L1.start
  constraint coincident P1 L1.end
  constraint coincident P2 L3.end
  constraint coincident P3 L4.end
  constraint coincident P5 L6.start
  constraint coincident P6 L8.start
  constraint coincident P7 L8.end
  constraint coincident P8 L9.end
  constraint coincident P9 L10.end
  constraint tangent L5 A0
  constraint tangent L7 A0
  constraint horizontal L11
  constraint vertical L12
  constraint horizontal L13
  constraint vertical L14
  constraint tangent L14 A2
  constraint tangent L11 A2
  constraint tangent L11 A3
  constraint tangent L12 A3
  constraint equal A2 A3
  constraint tangent L12 A4
  constraint tangent L13 A4
  constraint equal A2 A4
  constraint tangent L13 A5
  constraint tangent L14 A5
  constraint equal A2 A5
  constraint coincident L15 L19.start
  constraint coincident L15 L19.end
  constraint parallel L15 L19
  constraint perpendicular L10 L20
  constraint coincident P0 L0.start
  constraint perpendicular L0 L22
  constraint parallel L19 L24
  constraint parallel L19 L25
  constraint perpendicular L7 L23
  constraint coincident P49 P43
  measures "d78" radius of A0
  measures "d79" radius of A2
  measures "d80" distance of L14 L16
  measures "d91" distance of L19 L24
  measures "d92" distance of L15 L25
  measures "d93" distance of L12 L20
  measures "d94" distance of L13 L22
  measures "d102" distance of L12 L14
  measures "d103" distance of L7 L11
  measures "d104" distance of L11 L13
  measures "d105" distance of L7 L10
  measures "d106" distance of L0 L5
  measures "d109" distance of L22.end L24.end
  measures "d110" distance of L20.end L25.end
  measures "d111" distance of P9 L20.end
  measures "d112" distance of P0 L22.end
  measures "d113" distance of P8 P9
  measures "d114" distance of P0 L0.end
  measures "d115" distance of L25.end L85.end
  measures "d116" distance of L24.end L47.end
  measures "d117" distance of L67.end L99.end
  measures "d118" distance of L49.end L51.end
  measures "d119" diameter of A24
extrude "Extrude1" add sketch "Sketch2" along normal blind 80
move_body "Move1" bodies 1 to x (0, -1, 0) y (1, 0, 0) z (0, 0, 1) at (-3.4, 15.1, 15)
move_body "Move2" bodies 1 to x (1, 0, 0) y (0, 1, 0) z (0, 0, 1) at (3.4, 0, 0)
equation "d33 = ( 8.2 / 2 ) * 1 mm"
equation "d59 = ( 8.5 / 2 ) * 1 mm"
equation "d60 = ( 8.5 / 2 ) * 1 mm"
equation "d72 = ( 8.2 / 2 ) * 1 mm"
equation "Length = 80 mm"

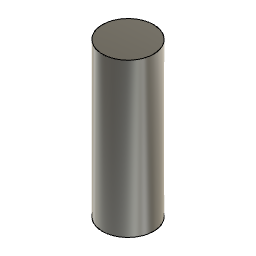
design "boggie_joint"
Autodesk Fusion 360 part; units mm, degrees
sketch "Sketch1" plane through (0, 0, 0) normal (0, 0, 1) x (1, 0, 0)
  circle A0 centre (0, 0) radius 8.325
  dimension "d1" = 16.65
  constraint coincident A0.centre origin
  measures "d1" diameter of A0
extrude "Extrude1" add sketch "Sketch1" along normal blind 50
equation "d1 = ( 8.325 * 2 ) * 1 mm"

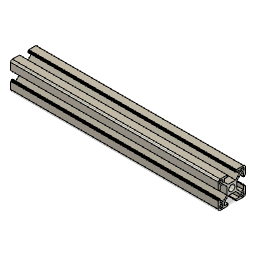
design "tslot_230mm"
Autodesk Fusion 360 part; units mm, degrees
sketch "Sketch1" plane through (0, 0, 0) normal (0, 1, 0) x (1, 0, 0)
  circle A0 centre (0, 0) radius 3.4
  line L0 (5.8, -4.25) -> (5.8, 4.25)
  line L1 (4.4302, 5.8) -> (-4.0698, 5.8)
  line L2 (-5.8, 4.25) -> (-5.8, -4.25)
  arc A1 (-13, 15) -> (-15, 13) centre (-13, 13) ccw
  arc A2 (15, 13) -> (13, 15) centre (13, 13) ccw
  arc A3 (12.9984, -15) -> (15, -13) centre (13, -13) ccw
  arc A4 (-15, -13.001) -> (-13, -15) centre (-13, -13) ccw
  line L3 (-9.0785, 8.25) -> (-13, 8.25)
  line L4 (-10.4448, -8.25) -> (-13, -8.25)
  line L5 (-8.25, 10.6606) -> (-8.25, 13)
  line L6 (8.25, 9.241) -> (8.25, 13)
  line L7 (-12.5, 9.75) -> (-10.75, 9.75)
  line L8 (-9.75, 10.75) -> (-9.75, 12.5)
  line L9 (-10.75, 13.5) -> (-12.5, 13.5)
  line L10 (-13.5, 12.5) -> (-13.5, 10.75)
  arc A5 (-12.5, 13.5) -> (-13.5, 12.5) centre (-12.5, 12.5) ccw
  arc A6 (-9.75, 12.5) -> (-10.75, 13.5) centre (-10.75, 12.5) ccw
  arc A7 (-10.75, 9.75) -> (-9.75, 10.75) centre (-10.75, 10.75) ccw
  arc A8 (-13.5, 10.75) -> (-12.5, 9.75) centre (-12.5, 10.75) ccw
  line L11 (-4.1, 14) -> (-5.1, 14)
  line L12 (-5.1, 14) -> (-5.1, 15)
  line L13 (4.1, 13) -> (4.1, 14)
  line L14 (4.1, 14) -> (5.1, 14)
  line L15 (5.1, 14) -> (5.1, 15)
  line L16 (-4.1, 14) -> (-4.1, 13)
  line L17 (0, 15) -> (0, -15) construction
  line L18 (-15, 0) -> (15, 0) construction
  line L19 (13.5, 12.5) -> (13.5, 10.75)
  line L20 (12.5, 9.75) -> (10.75, 9.75)
  arc A9 (10.75, 13.5) -> (9.75, 12.5) centre (10.75, 12.5) ccw
  arc A10 (9.75, 10.75) -> (10.75, 9.75) centre (10.75, 10.75) ccw
  line L21 (9.75, 10.75) -> (9.75, 12.5)
  arc A11 (12.5, 9.75) -> (13.5, 10.75) centre (12.5, 10.75) ccw
  line L22 (10.75, 13.5) -> (12.5, 13.5)
  arc A12 (13.5, 12.5) -> (12.5, 13.5) centre (12.5, 12.5) ccw
  arc A13 (-9.75, -10.75) -> (-10.75, -9.75) centre (-10.75, -10.75) ccw
  line L23 (-9.75, -10.75) -> (-9.75, -12.5)
  line L24 (-13.5, -12.5) -> (-13.5, -10.75)
  line L25 (-10.75, -13.5) -> (-12.5, -13.5)
  arc A14 (-13.5, -12.5) -> (-12.5, -13.5) centre (-12.5, -12.5) ccw
  line L26 (-12.5, -9.75) -> (-10.75, -9.75)
  arc A15 (-12.5, -9.75) -> (-13.5, -10.75) centre (-12.5, -10.75) ccw
  arc A16 (-10.75, -13.5) -> (-9.75, -12.5) centre (-10.75, -12.5) ccw
  arc A17 (12.5, -13.5) -> (13.5, -12.5) centre (12.5, -12.5) ccw
  arc A18 (10.75, -9.75) -> (9.75, -10.75) centre (10.75, -10.75) ccw
  arc A19 (9.75, -12.5) -> (10.75, -13.5) centre (10.75, -12.5) ccw
  line L27 (9.75, -10.75) -> (9.75, -12.5)
  line L28 (12.5, -9.75) -> (10.75, -9.75)
  arc A20 (13.5, -10.75) -> (12.5, -9.75) centre (12.5, -10.75) ccw
  line L29 (13.5, -12.5) -> (13.5, -10.75)
  line L30 (10.75, -13.5) -> (12.5, -13.5)
  line L31 (-4.1, -14) -> (-5.1, -14)
  line L32 (-4.1, -14) -> (-4.1, -13)
  line L33 (-5.1, -14) -> (-5.1, -15)
  line L34 (4.1, -13) -> (4.1, -14)
  line L35 (4.1, -14) -> (5.1, -14)
  line L36 (5.1, -14) -> (5.1, -15)
  line L37 (-8.25, -10.6606) -> (-8.25, -13)
  line L38 (-13, -15) -> (-5.1, -15)
  line L39 (5.1, -15) -> (12.9984, -15)
  line L40 (-8.25, -13) -> (-4.1, -13)
  line L41 (13, 15) -> (5.1, 15)
  line L42 (-5.1, 15) -> (-13, 15)
  line L43 (8.25, 13) -> (4.1, 13)
  line L44 (-4.1, 13) -> (-8.25, 13)
  line L45 (8.25, -9.768) -> (8.25, -13)
  line L46 (-13, -13) -> (12.5, 12.5) construction
  line L47 (-12.5, 12.5) -> (13, -13) construction
  line L48 (13, -8.25) -> (9.8438, -8.25)
  line L49 (5.8, -4.25) -> (9.8438, -8.25)
  line L50 (4.1, -13) -> (8.25, -13)
  line L51 (13, 8.25) -> (9.3051, 8.25)
  line L52 (-4.2601, -5.7908) -> (4.2399, -5.7908)
  line L53 (-13, 4.1) -> (-14, 4.1)
  line L54 (-14, 4.1) -> (-14, 5.1)
  line L55 (-14, 5.1) -> (-15, 5.1)
  line L56 (-13, -4.1) -> (-14, -4.1)
  line L57 (-14, -4.1) -> (-14, -5.1)
  line L58 (-14, -5.1) -> (-15, -5.1)
  line L59 (-13, 8.25) -> (-13, 4.1)
  line L60 (-13, -4.1) -> (-13, -8.25)
  line L61 (-15, 13) -> (-15, 5.1)
  line L62 (-15, -5.1) -> (-15, -13.001)
  line L63 (13, -8.25) -> (13, -3.9838)
  line L64 (13, 4.0895) -> (13, 10.5589)
  line L65 (15, -13) -> (15, -4.9838)
  line L66 (15, 5.0895) -> (15, 13)
  point P0 (15, -15)
  point P1 (15, 15)
  point P2 (-15, 15)
  point P3 (13, 13)
  point P4 (-13, -13)
  point P5 (13, -13)
  point P6 (13, -13)
  point P7 (13, -10.5589)
  dimension "d1" = 6.8
  dimension "d2" = 30
  dimension "d3" = 30
  dimension "d5" = 9.2
  dimension "d6" = 9.2
  dimension "d7" = 9.2
  dimension "d13" = 2
  dimension "d14" = 2
  dimension "d15" = 2
  dimension "d16" = 2
  dimension "d17" = 16.5
  dimension "d19" = 16.5
  dimension "d22" = 1.5
  dimension "d23" = 1.5
  dimension "d24" = 1.5
  dimension "d25" = 1.5
  dimension "d26" = 1
  dimension "d33" = 4.1
  dimension "d34" = 1
  dimension "d35" = 2
  dimension "d36" = 2
  dimension "d37" = 2
  dimension "d39" = 3.75
  dimension "d40" = 3.75
  dimension "d41" = 5.8
  dimension "d42" = 5.8
  dimension "d43" = 5.8
  dimension "d45" = 8.5
  dimension "d46" = 8.5
  dimension "d48" = 8.5
  dimension "d49" = 1
  dimension "d51" = 8.2
  dimension "d52" = 1.5
  dimension "d53" = 1.5
  dimension "d54" = 1.5
  dimension "d55" = 1.5
  dimension "d57" = 1.5
  dimension "d58" = 1.5
  dimension "d59" = 4.25
  dimension "d60" = 4.25
  dimension "d64" = 8.5
  dimension "d65" = 1
  dimension "d66" = 1
  dimension "d67" = 1
  dimension "d68" = 1
  dimension "d71" = 8.2
  dimension "d72" = 4.1
  constraint horizontal L38
  constraint vertical L65
  constraint horizontal L41
  constraint vertical L61
  constraint vertical L0
  constraint horizontal L1
  constraint vertical L2
  constraint coincident P2 L61
  constraint coincident P2 L41
  constraint tangent A1 L61
  constraint coincident P1 L41
  constraint coincident P1 L65
  constraint tangent A2 L41
  constraint coincident P0 L38
  constraint coincident P0 L65
  constraint tangent A3 L65
  constraint tangent A4 L38
  constraint parallel L63 L65
  constraint horizontal L7
  constraint vertical L8
  constraint horizontal L9
  constraint vertical L10
  constraint tangent L10 A5
  constraint tangent L9 A5
  constraint tangent L9 A6
  constraint tangent L8 A6
  constraint equal A5 A6
  constraint tangent L8 A7
  constraint tangent L7 A7
  constraint equal A5 A7
  constraint tangent L7 A8
  constraint tangent L10 A8
  constraint equal A5 A8
  constraint perpendicular L12 L41
  constraint perpendicular L13 L43
  constraint perpendicular L13 L14
  constraint perpendicular L15 L41
  constraint coincident L16.end L43
  constraint perpendicular L16 L43
  constraint symmetric A1.centre L17 P3
  constraint symmetric L10.start L17 L19.start
  constraint symmetric L9.end L17 L22.end
  constraint symmetric A5 L17 A12
  constraint symmetric L9.start L17 A9.start
  constraint symmetric L8.end L17 A9.end
  constraint symmetric A6 L17 A9
  constraint symmetric L8.start L17 A10.start
  constraint symmetric L7.end L17 L20.end
  constraint symmetric A7 L17 A10
  constraint symmetric L7.start L17 L20.start
  constraint symmetric L10.end L17 L19.end
  constraint symmetric A8 L17 A11
  constraint symmetric P3 L18 P6
  constraint symmetric L64.end L18 P7
  constraint symmetric L18 L19.end A20.start
  constraint symmetric L18 L20.end A18.start
  constraint symmetric L18 P3 P6
  constraint symmetric L18 L19.start A17.end
  constraint symmetric L18 L22.end A17.start
  constraint symmetric L18 A9.end A19.start
  constraint symmetric L18 L20.start L28.start
  constraint symmetric L18 A10.start A18.end
  constraint symmetric L18 A9.start A19.end
  constraint symmetric L18 A9 A19
  constraint symmetric L18 A10 A18
  constraint symmetric L18 A11 A20
  constraint symmetric L18 A12 A17
  constraint symmetric L5.end L18 L37.end
  constraint symmetric L11.start L18 L31.start
  constraint symmetric L11.end L18 L31.end
  constraint symmetric L12.end L18 L33.end
  constraint symmetric L13.start L18 L34.start
  constraint symmetric L13.end L18 L34.end
  constraint symmetric L14.end L18 L35.end
  constraint symmetric L15.end L18 L36.end
  constraint symmetric L16.end L18 L32.end
  constraint collinear L38 L39
  constraint collinear L41 L42
  constraint collinear L43 L44
  constraint symmetric L17 L37.end L45.end
  constraint coincident P4 A4.centre
  constraint coincident A12.centre L46.end
  constraint coincident A5.centre L47.start
  constraint coincident P6 P5
  constraint perpendicular L48 L63
  constraint vertical L45
  constraint coincident L51.start L63
  constraint horizontal L52
  constraint coincident L56.start L59
  constraint coincident L58.end L61
  constraint collinear L59 L60
  constraint collinear L61 L62
  constraint perpendicular L53 L54
  constraint perpendicular L54 L55
  constraint perpendicular L57 L58
  constraint perpendicular L56 L57
  constraint perpendicular L58 L62
  constraint collinear L65 L66
  measures "d1" diameter of A0
  measures "d2" distance of P0 P1
  measures "d3" distance of P1 P2
  measures "d5" distance of L0 L65
  measures "d6" distance of L2 L61
  measures "d7" distance of L1 L41
  measures "d13" radius of A1
  measures "d14" radius of A2
  measures "d15" radius of A3
  measures "d16" radius of A4
  measures "d17" distance of L3 L4
  measures "d19" distance of L5 L6
  measures "d22" distance of L5 L8
  measures "d23" distance of L10 L61
  measures "d24" distance of L3 L7
  measures "d25" distance of L9 L41
  measures "d26" radius of A5
  measures "d33" distance of A0.centre L13
  measures "d34" distance of L11.start L11.end
  measures "d35" distance of L41 L43
  measures "d36" distance of L59 L61
  measures "d37" distance of L63 L65
  measures "d39" distance of L8 L10
  measures "d40" distance of L7 L9
  measures "d41" distance of A0.centre L1
  measures "d42" distance of A0.centre L2
  measures "d43" distance of A0.centre L0
  measures "d45" distance of L1.end L1.start
  measures "d46" distance of L2.start L2.end
  measures "d48" distance of L0.start L0.end
  measures "d49" distance of L13.end L14.end
  measures "d51" distance of L13 L16
  measures "d52" distance of L23 L37
  measures "d53" distance of L4 L26
  measures "d54" distance of L27 L45
  measures "d55" distance of L28 L48
  measures "d57" distance of L20 L51
  measures "d58" distance of L6 L21
  measures "d59" distance of L2.end L18
  measures "d60" distance of L0.start L18
  measures "d64" distance of L52.start L52.end
  measures "d65" distance of L53.end L54.end
  measures "d66" distance of L53.start L53.end
  measures "d67" distance of L56.start L56.end
  measures "d68" distance of L56.end L57.end
  measures "d71" distance of L53 L56
  measures "d72" distance of L18 L53